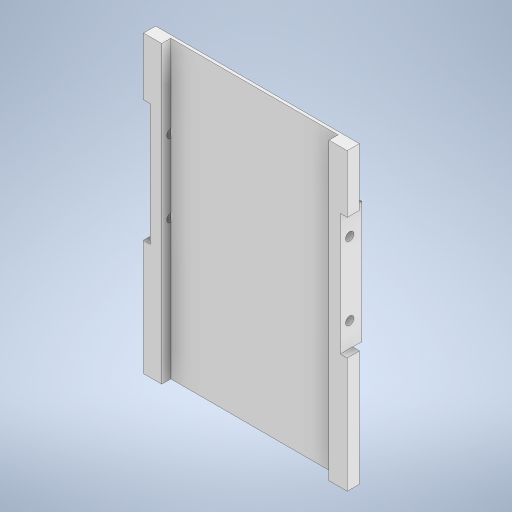
# Autodesk Inventor part: cover_right
Saved by Autodesk Inventor 2024.1 (Build 281209000, 209)
## iProperties
Created: 2025-03-07
Part Number: cover_right
Material: 一般
Document SubType Name: モデリング
Designer: hibik
Density: 1 g/cm^3
Appearance: 既定
Sheet Metal Rule: Default
Author: hibik
Autodesk Inventor part; units mm, degrees
ref_plane "YZ Plane" through (0, 0, 0) normal (1, 0, 0) x (0, 1, 0)
ref_plane "XZ Plane" through (0, 0, 0) normal (0, 1, 0) x (-1, 0, 0)
ref_plane "XY Plane" through (0, 0, 0) normal (0, 0, 1) x (1, 0, 0)
sketch "スケッチ1" plane through (0, 0, 0) normal (0, 0, 1) x (1, 0, 0)
  line L0 (33.5, -48.5) -> (-33.5, -48.5)
  line L1 (-33.5, -48.5) -> (-33.5, 48.5)
  line L2 (-33.5, 48.5) -> (33.5, 48.5)
  line L3 (33.5, 48.5) -> (33.5, -48.5)
  line L4 (33.5, -48.5) -> (-33.5, 48.5) construction
  line L5 (-33.5, -48.5) -> (33.5, 48.5) construction
  point P0 (0, 0)
  dimension "d0" = 67
  dimension "d1" = 97
  constraints: 12 end point, 2 midpoint, 2 parallel, 1 horizontal, 1 perpendicular
  measures "d0" distance of L1.end L2.end
  measures "d1" distance of L0.end L1.end
extrude "押し出し1" add sketch "スケッチ1" along normal blind 1
sketch "スケッチ3" plane through (33.5, -48.5, 0) normal (1, 0, 0) x (0, 0, -1)
  line L0 (0, 78) -> (-5, 78)
  line L1 (-5, 78) -> (-5, 38)
  line L2 (-5, 38) -> (0, 38)
  line L3 (0, 38) -> (0, 78)
  circle A0 centre (-1, 70) radius 1.35
  line L4 (0, 97) -> (-1, 97) projected
  line L5 (0, 0) -> (0, 97) projected
  circle A1 centre (-1, 46) radius 1.35
  point P0 (0, 48.5)
  dimension "d4" = 5
  dimension "d5" = 27
  dimension "d6" = 8
  dimension "d7" = 40
  dimension "d8" = 2.7
  dimension "d9" = 8
  dimension "d48" = 1
  constraints: 8 end point, 2 centre point, 2 parallel, 1 collinear, 1 equal radius, 1 horizontal, 1 perpendicular, 1 vertical alignment
  measures "d4" distance of L0.start L0.end
  measures "d5" distance from line of L4 A0.centre
  measures "d6" distance from line of L0 A0.centre
  measures "d7" distance of L0.end L1.end
  measures "d8" diameter of A0
  measures "d9" distance from line of L2 A1.centre
  measures "d48" distance from line of L3 A0.centre
extrude "押し出し2" add sketch "スケッチ3" against normal blind 6 contours L3 A0 A1 L2 L1 L0
extrude "押し出し3" cut sketch "スケッチ3" against normal blind 2.2 contours L3 A0 A1 L2 L1 L0
mirror "ミラー1" about plane through (0, 0, 0) normal (1, 0, 0) of "押し出し2", "押し出し3"
sketch "スケッチ12" plane through (31.3, -48.5, 0) normal (1, 0, 0) x (0, 0, -1)
  line L0 (-1, 78) -> (-5, 78) projected
  line L1 (-5, 78) -> (3, 78)
  line L2 (3, 78) -> (3, 38)
  line L3 (3, 38) -> (-5, 38)
  line L4 (-5, 38) -> (-5, 78)
  arc A0 (-1, 71.35) -> (-1, 68.65) centre (-1, 70) ccw projected
  arc A1 (-1, 47.35) -> (-1, 44.65) centre (-1, 46) ccw projected
  circle A2 centre (-1, 70) radius 1.35
  circle A3 centre (-1, 46) radius 1.35
  point P0 (0, 48.5)
  point P1 (0, 38)
  point P2 (-1, 68.65)
  point P3 (-1, 44.65)
  dimension "d49" = 8
  constraints: 8 end point, 2 centre point, 2 coincident, 2 concentric, 2 parallel, 1 horizontal, 1 perpendicular, 1 point on line
  measures "d49" distance of L0.end L1.end
extrude "押し出し15" add sketch "スケッチ12" against normal up to surface (3.8 mm away)
sketch "スケッチ13" plane through (27.5, -10.5, -3) normal (-1, 0, 0) x (0, 0, 1)
  line L0 (4, 30.65) -> (4, 33.35) projected
  circle A0 centre (4, 32) radius 1.35
  line L1 (4, 6.65) -> (4, 9.35) projected
  circle A1 centre (4, 8) radius 1.35
  arc A2 (4, 30.65) -> (4, 33.35) centre (4, 32) ccw projected
  arc A3 (4, 6.65) -> (4, 9.35) centre (4, 8) ccw projected
  point P0 (3, 10.5)
  constraints: 2 centre point, 2 concentric, 2 midpoint
extrude "押し出し16" cut sketch "スケッチ13" against normal through all
mirror "ミラー2" about plane through (0, 0, 0) normal (1, 0, 0) of "押し出し15", "押し出し16"
sketch "スケッチ14" plane through (0, 0, 1) normal (0, 0, 1) x (1, 0, 0)
  line L0 (-27.5, -10.5) -> (-27.5, 29.5) projected
  line L1 (27.5, -10.5) -> (27.5, 29.5) projected
  line L2 (33.5, 48.5) -> (-33.5, 48.5) projected
  line L3 (-33.5, -48.5) -> (33.5, -48.5) projected
  line L4 (-27.5, 48.5) -> (27.5, 48.5)
  line L5 (27.5, 48.5) -> (27.5, -48.5)
  line L6 (27.5, -48.5) -> (-27.5, -48.5)
  line L7 (-27.5, -48.5) -> (-27.5, 48.5)
  line L8 (-27.5, 22.85) -> (-27.5, 20.15) projected
  line L9 (-27.5, 20.15) -> (-27.5, -1.15) projected
  line L10 (-27.5, -1.15) -> (-27.5, -3.85) projected
  line L11 (-27.5, -3.85) -> (-27.5, -10.5) projected
  line L12 (-27.5, -10.5) -> (-31.3, -10.5) projected
  line L13 (-31.3, -10.5) -> (-33.5, -10.5) projected
  line L14 (-33.5, -10.5) -> (-33.5, -48.5) projected
  line L15 (-33.5, -48.5) -> (33.5, -48.5) projected
  line L16 (33.5, -48.5) -> (33.5, -10.5) projected
  line L17 (33.5, -10.5) -> (31.3, -10.5) projected
  line L18 (31.3, -10.5) -> (27.5, -10.5) projected
  line L19 (27.5, -10.5) -> (27.5, -3.85) projected
  line L20 (27.5, -3.85) -> (27.5, -1.15) projected
  line L21 (27.5, -1.15) -> (27.5, 20.15) projected
  line L22 (27.5, 20.15) -> (27.5, 22.85) projected
  line L23 (27.5, 22.85) -> (27.5, 29.5) projected
  line L24 (27.5, 29.5) -> (31.3, 29.5) projected
  line L25 (31.3, 29.5) -> (33.5, 29.5) projected
  line L26 (33.5, 29.5) -> (33.5, 48.5) projected
  line L27 (33.5, 48.5) -> (-33.5, 48.5) projected
  line L28 (-33.5, 48.5) -> (-33.5, 29.5) projected
  line L29 (-33.5, 29.5) -> (-31.3, 29.5) projected
  line L30 (-31.3, 29.5) -> (-27.5, 29.5) projected
  line L31 (-27.5, 29.5) -> (-27.5, 22.85) projected
  point P0 (0, 0)
  point P1 (-27.5, -48.5)
  constraints: 8 end point, 2 collinear, 2 parallel, 2 point on line, 1 horizontal, 1 perpendicular
extrude "押し出し17" add sketch "スケッチ14" along normal up to surface (4 mm away) contours L7 L3 L14 L13 L12 | L5 L18 L17 L16 L3 | L30 L29 L28 L2 L7 | L2 L26 L25 L24 L5
sketch "スケッチ15" plane through (-33.5, -48.5, 5) normal (0, 0, 1) x (1, 0, 0)
  line L0 (2.2, 78) -> (2.2, 38) projected
  line L1 (0, 38) -> (2.2, 38) projected
  line L2 (0, 0) -> (0, 38) projected
  line L3 (6, 0) -> (0, 0) projected
  line L4 (6, 97) -> (6, 0) projected
  line L5 (0, 97) -> (6, 97) projected
  line L6 (0, 78) -> (0, 97) projected
  line L7 (2.2, 78) -> (0, 78) projected
  line L8 (64.8, 38) -> (64.8, 78) projected
  line L9 (67, 78) -> (64.8, 78) projected
  line L10 (67, 97) -> (67, 78) projected
  line L11 (61, 97) -> (67, 97) projected
  line L12 (61, 0) -> (61, 97) projected
  line L13 (67, 0) -> (61, 0) projected
  line L14 (67, 38) -> (67, 0) projected
  line L15 (64.8, 38) -> (67, 38) projected
  point P0 (33.5, 48.5)
extrude "押し出し18" cut sketch "スケッチ15" against normal blind 1
equation "\"d9\" = d6"
equation "\"BendRadius\" = Thickness"
equation "\"BendReliefWidth\" = Thickness"
equation "\"BendReliefDepth\" = 0.5 * Thickness"
equation "\"CornerReliefSize\" = 4 * Thickness"
equation "\"MinimumRemnant\" = 2 * Thickness"
equation "\"TransitionRadius\" = BendRadius"
equation "\"JacobiRadiusSize\" = BendRadius"
equation "\"GapSize\" = Thickness"
equation "\"Thickness\" = 3.048"
